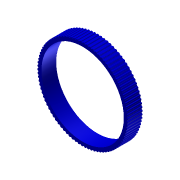
# Autodesk Inventor part: Nitrile Tread 6in
Saved by Autodesk Inventor 2011 (Build 150239000, 239)
## iProperties
Created: 2012-06-01
Part Number: Nitrile Tread 6in
Document SubType Name: Modeling
Designer: Nemo
Density: 1.3551 g/cm^3
Material: Rubber
Mass: 102.058 g
Surface Area: 329.584 cm^2
Volume: 75.3141 cm^3
Author: Nemo
Autodesk Inventor part; units mm, degrees
ref_plane "YZ Plane" through (0, 0, 0) normal (1, 0, 0) x (0, 1, 0)
ref_plane "XZ Plane" through (0, 0, 0) normal (0, 1, 0) x (-1, 0, 0)
ref_plane "XY Plane" through (0, 0, 0) normal (0, 0, 1) x (1, 0, 0)
sketch "Sketch1" plane through (0, 0, 0) normal (0, 0, 1) x (1, 0, 0)
  circle A0 centre (0, 0) radius 71.12
  circle A1 centre (0, 0) radius 76.835
  dimension "d0" = 142.24
  dimension "d1" = 153.67
  constraints: 2 centre point, 2 coincident
  measures "d0" diameter of A0
  measures "d1" diameter of A1
extrude "Extrusion1" add sketch "Sketch1" along normal blind 25.4
sketch "Sketch2" plane through (0, 0, 25.4) normal (0, 0, 1) x (1, 0, 0)
  circle A0 centre (0, 0) radius 76.835 projected
  line L0 (0, 0) -> (0, 76.835) construction
  line L1 (0, 0) -> (0, 76.835) construction
  line L2 (0, 0) -> (0, 76.835) construction
  line L3 (2.6815, 76.7882) -> (0, 0) construction
  arc A1 (2.6815, 76.7882) -> (0, 76.835) centre (0, 0) ccw
  line L4 (0, 76.835) -> (0, 77.4674)
  line L5 (2.6815, 76.7882) -> (2.7036, 77.4202)
  arc A2 (2.0859, 78.0771) -> (0.6402, 78.1024) centre (0, 0) ccw
  arc A3 (0.6402, 78.1024) -> (0, 77.4674) centre (0.635, 77.4674) ccw
  arc A4 (2.7036, 77.4202) -> (2.0859, 78.0771) centre (2.069, 77.4424) ccw
  line L6 (0, 0) -> (5.3597, 76.6478) construction
  arc A5 (4.7313, 76.6892) -> (3.3108, 76.7636) centre (0, 0) ccw
  arc A6 (2.7036, 77.4202) -> (3.3108, 76.7636) centre (3.3382, 77.398) ccw
  line L7 (5.3597, 76.6478) -> (5.4039, 77.2787)
  arc A7 (4.7313, 76.6892) -> (5.4039, 77.2787) centre (4.7704, 77.323) ccw
  point P0 (0, 78.105)
  point P1 (2.7258, 78.0574)
  dimension "d4" = 2
  dimension "d7" = 1.27
  dimension "d8" = 0.635
  dimension "d10" = 2
  dimension "d11" = 0.635
  dimension "d12" = 0.635
  constraints: 16 end point, 16 point on circle, 8 tangent, 7 centre point, 3 coincident, 3 collinear, 3 point on line, 1 equal length, 1 equal radius, 1 vertical, 8 other
  measures "d4" angle of L2 L3
  measures "d8" radius of A3
  measures "d10" angle of L3 L6
  measures "d11" radius of A6
  measures "d12" radius of A7
extrude "Extrusion2" add sketch "Sketch2" against normal up to surface (25.4 mm away) contours A0 A7 L7 | L4 A3 A2 A4 L5 A0 | L5 A6 A0
pattern_circular "Circular Pattern1" count 90 over 360 about axis through (0, 0, 0) along (0, 0, 1) of "Extrusion2"
equation "\"d10\" = d4"
equation "\"d11\" = d8"
equation "\"d12\" = d8"
body "Solid1"
